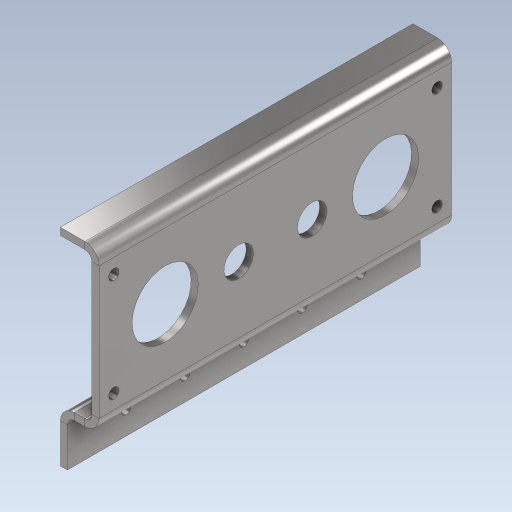
# Autodesk Inventor part: CH-1-01-GearboxHousingMotorSide
Saved by Autodesk Inventor 2023 (Build 270158000, 158)
## iProperties
Created: 2023-02-02
Part Number: CH-1-01-GearboxHousingMotorSide
Material: Steel, Alloy
Document SubType Name: Sheet Metal
Designer: Dave
Density: 7.73 g/cm^3
Sheet Metal Rule: Default
Appearance: Semi-Polished
Author: Dave
Autodesk Inventor part; units mm, degrees
ref_plane "YZ Plane" through (0, 0, 0) normal (1, 0, 0) x (0, 1, 0)
ref_plane "XZ Plane" through (0, 0, 0) normal (0, 1, 0) x (-1, 0, 0)
ref_plane "XY Plane" through (0, 0, 0) normal (0, 0, 1) x (1, 0, 0)
sketch "Sketch3" plane through (-13.672, 63.246, 0) normal (0, 1, 0) x (1, 0, 0)
  line L0 (10.624, 0) -> (10.624, 152.4) projected
  line L1 (0, 152.4) -> (10.624, 152.4) projected
  line L2 (0, 0) -> (0, 152.4) projected
  line L3 (10.624, 0) -> (0, 0) projected
  point P0 (13.672, 0)
  point P1 (5.312, 127)
  point P2 (5.312, 152.4)
  point P3 (5.312, 101.6)
  point P4 (5.312, 76.2)
  point P5 (5.312, 50.8)
  point P6 (5.312, 25.4)
  dimension "d28" = 25.4
  dimension "d31" = 25.4
  constraints: 1 midpoint, 1 vertical, 1 vertical alignment, 4 other
  measures "d28" distance from line of L1 point (5.312, 127)
  measures "d31" distance of point (5.312, 127) point (5.312, 101.6)
sketch "Sketch1" plane through (0, 0, 0) normal (1, 0, 0) x (0, 1, 0)
  line L0 (0, 0) -> (57.15, 0)
  line L1 (57.15, 0) -> (57.15, -152.4)
  line L2 (57.15, -152.4) -> (0, -152.4)
  line L3 (0, -152.4) -> (0, 0)
  circle A0 centre (28.575, -28.575) radius 14.2875
  circle A1 centre (28.575, -60.325) radius 6.35
  circle A2 centre (28.575, -92.075) radius 6.35
  circle A3 centre (28.575, -123.825) radius 14.2875
  circle A4 centre (50.8, -6.35) radius 2.2479
  circle A5 centre (50.8, -146.05) radius 2.2479
  circle A6 centre (6.35, -146.05) radius 2.2479
  circle A7 centre (6.35, -6.35) radius 2.2479
  line L4 (50.8, -6.35) -> (6.35, -6.35) construction
  line L5 (6.35, -6.35) -> (6.35, -146.05) construction
  line L6 (6.35, -146.05) -> (50.8, -146.05) construction
  line L7 (50.8, -146.05) -> (50.8, -6.35) construction
  line L8 (57.15, 0) -> (69.85, 0)
  line L9 (69.85, 0) -> (69.85, -152.4)
  line L10 (69.85, -152.4) -> (57.15, -152.4)
  line L11 (57.15, -152.4) -> (57.15, 0)
  line L12 (0, -152.4) -> (-12.7, -152.4)
  line L13 (-12.7, -152.4) -> (-12.7, 0)
  line L14 (-12.7, 0) -> (0, 0)
  line L15 (0, 0) -> (0, -152.4)
  line L16 (28.575, -123.825) -> (28.575, -28.575)
  point P0 (28.575, -152.4)
  point P1 (28.575, -6.35)
  point P2 (28.575, 0)
  point P3 (50.8, -76.2)
  point P4 (57.15, -76.2)
  point P5 (57.15, -76.2)
  point P6 (28.575, -76.2)
  dimension "d0" = 57.15
  dimension "d1" = 152.4
  dimension "d2" = 31.75
  dimension "d3" = 31.75
  dimension "d4" = 31.75
  dimension "d6" = 28.575
  dimension "d7" = 12.7
  dimension "d8" = 28.575
  dimension "d11" = 4.4958
  dimension "d12" = 139.7
  dimension "d13" = 44.45
  dimension "d14" = 12.7
  dimension "d15" = 152.4
  dimension "d16" = 12.7
  dimension "d17" = 152.4
  measures "d0" distance of L1.end L2.end
  measures "d1" distance of L0.end L1.end
  measures "d2" distance of A1.centre L16.end
  measures "d3" distance of A2.centre A1.centre
  measures "d4" distance of L16.start A2.centre
  measures "d6" diameter of A0
  measures "d7" diameter of A1
  measures "d8" diameter of A3
  measures "d11" diameter of A4
  measures "d12" distance of L6.end L4.start
  measures "d13" distance of L4.start L4.end
  measures "d14" distance of L9.end L10.end
  measures "d15" distance of L8.end L9.end
  measures "d16" distance of L13.end L14.end
  measures "d17" distance of L12.end L13.end
extrude "Plate2" add sketch "Sketch1" along normal blind 3.048 contours L0 L1 L2 L3
sketch "Sketch2" plane through (-3.048, 60.198, -152.4) normal (0, 1, 0) x (-1, 0, 0)
  line L0 (0, 152.4) -> (0, 0)
  line L1 (0, 0) -> (10.624, 0)
  line L2 (10.624, 0) -> (10.624, 152.4)
  line L3 (10.624, 152.4) -> (0, 152.4)
  constraints: 6 end point, 1 horizontal, 1 perpendicular, 1 vertical
edge flange "Flange1" height 16.72 angle 90 thickness 3.048 bend radius 3.048 thickness toward (0, 1, 0) relief tear relief width 3.048 relief depth 1.524 corner gap 3.048 corner form 0 edges at (0, 57.15, -76.2) (0, 0, -76.2) wall of the first edge with corners at (-3.048, 60.198, 0) (-3.048, 60.198, -152.4) (-13.672, 60.198, -152.4) (-13.672, 60.198, 0)
bend "Bend1"
corner "Corner1"
sketch "Sketch4" plane through (-10.624, -3.048, -152.4) normal (-1, 0, 0) x (0, -1, 0)
  line L0 (0, 152.4) -> (0, 0)
  line L1 (0, 0) -> (23.048, 0)
  line L2 (23.048, 0) -> (23.048, 152.4)
  line L3 (23.048, 152.4) -> (0, 152.4)
  constraints: 6 end point, 1 horizontal, 1 perpendicular, 1 vertical
edge flange "Flange2" height 20 angle 90 thickness 3.048 bend radius 3.048 thickness toward (-1, 0, 0) relief tear relief width 3.048 relief depth 1.524 edges at (-13.672, -6.096, -76.2) wall of the first edge with corners at (-10.624, -3.048, 0) (-10.624, -3.048, -152.4) (-10.624, -26.096, -152.4) (-10.624, -26.096, 0)
bend "Bend2"
corner "Corner2"
sketch "Sketch5" plane through (-10.624, -26.096, 0) normal (1, 0, 0) x (0, 0, -1)
  line L0 (152.4, 16.952) -> (152.4, 0) projected
  line L1 (0, 0) -> (152.4, 0) projected
  point P0 (0, 26.096)
  point P1 (127, 10)
  point P2 (101.6, 10)
  point P3 (76.2, 10)
  point P4 (50.8, 10)
  point P5 (25.4, 10)
  dimension "d53" = 25.4
  dimension "d54" = 10
  dimension "d57" = 25.4
  constraints: 1 horizontal, 4 other
  measures "d53" distance from line of L0 point (127, 10)
  measures "d54" distance from line of L1 point (127, 10)
  measures "d57" distance of point (127, 10) point (101.6, 10)
hole "Hole2" at (-10.624, -16.096, -127) at (-10.624, -16.096, -101.6) at (-10.624, -16.096, -76.2) at (-10.624, -16.096, -50.8) at (-10.624, -16.096, -25.4) direction (-1, 0, 0) diameter 4.134 end through all
equation "\"d10\" = Thickness"
equation "\"d18\" = BendReliefWidth"
equation "\"d19\" = BendReliefDepth"
equation "\"d20\" = MinimumRemnant"
equation "\"d21\" = TransitionRadius"
equation "\"d24\" = BendRadius"
equation "\"d25\" = CornerReliefSize"
equation "\"d26\" = GapSize"
equation "\"d27\" = JacobiRadiusSize"
equation "\"d43\" = BendReliefWidth"
equation "\"d44\" = BendReliefDepth"
equation "\"d45\" = MinimumRemnant"
equation "\"d46\" = TransitionRadius"
equation "\"d49\" = BendRadius"
equation "\"d50\" = CornerReliefSize"
equation "\"d51\" = GapSize"
equation "\"d52\" = JacobiRadiusSize"
equation "\"BendRadius\" = Thickness"
equation "\"BendReliefWidth\" = Thickness"
equation "\"BendReliefDepth\" = 0.5 * Thickness"
equation "\"CornerReliefSize\" = 4 * Thickness"
equation "\"MinimumRemnant\" = 2 * Thickness"
equation "\"TransitionRadius\" = BendRadius"
equation "\"JacobiRadiusSize\" = BendRadius"
equation "\"GapSize\" = Thickness"
equation "\"Thickness\" = 3.048"
body "Solid2"
